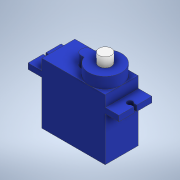
# Autodesk Inventor part: MicroServo
Saved by Autodesk Inventor 2021 (Build 250183000, 183)
## iProperties
Created: 2020-12-16
Part Number: MicroServo
Material: Generisch
Document SubType Name: Modeling
Designer: laure
Density: 1 g/cm^3
Appearance: Vorgabe
Author: laure
Autodesk Inventor part; units mm, degrees
ref_plane "YZ Plane" through (0, 0, 0) normal (1, 0, 0) x (0, 1, 0)
ref_plane "XZ Plane" through (0, 0, 0) normal (0, 1, 0) x (-1, 0, 0)
ref_plane "XY Plane" through (0, 0, 0) normal (0, 0, 1) x (1, 0, 0)
sketch "Skizze1" plane through (0, 0, 0) normal (0, 0, 1) x (1, 0, 0)
  line L0 (-11.5, 11) -> (11.5, 11)
  line L1 (11.5, 11) -> (11.5, -11)
  line L2 (11.5, -11) -> (-11.5, -11)
  line L3 (-11.5, -11) -> (-11.5, 11)
  line L4 (0, -15.4) -> (0, 15.4) projected
  line L5 (-23.1, 0) -> (23.1, 0) projected
  line L6 (-11.5, 7) -> (-16.5, 7)
  line L7 (-16.5, 7) -> (-16.5, 5)
  line L8 (-16.5, 5) -> (-11.5, 5)
  line L9 (-11.5, 5) -> (-11.5, 7)
  line L10 (11.5, 7) -> (16.5, 7)
  line L11 (16.5, 7) -> (16.5, 5)
  line L12 (16.5, 5) -> (11.5, 5)
  line L13 (11.5, 5) -> (11.5, 7)
  point P0 (0, 0)
  dimension "d0" = 23
  dimension "d1" = 22
  dimension "d2" = 16
  dimension "d3" = 2
  dimension "d4" = 5
  constraints: 24 end point, 4 parallel, 4 symmetric about line, 2 horizontal, 2 perpendicular, 1 point on line, 2 other
  measures "d0" distance between parallel lines of L1 L3
  measures "d1" distance between parallel lines of L2 L0
  measures "d2" distance between parallel lines of L8 L2
  measures "d3" distance between parallel lines of L6 L8
  measures "d4" distance between parallel lines of L7 L3
extrude "Extrusion1" add sketch "Skizze1" against normal mid plane 12 contours L0 L4 L5 L3 | L0 L1 L5 L4 | L5 L1 L2 L4 | L4 L2 L3 L5
extrude "Extrusion2" add sketch "Skizze1" along normal mid plane 12 contours L3 L8 L7 L6 | L10 L11 L12 L1
sketch "Skizze2" plane through (-11.5, 11, -6) normal (0, 1, 0) x (1, 0, 0)
  arc A0 (11.3431, -8) -> (11.3431, -4) centre (17, -6) ccw
  line L0 (0, 0) -> (23, 0) projected
  line L1 (23, 0) -> (23, -12) projected
  arc A1 (10.2601, -4) -> (10.2601, -8) centre (10.2601, -6) ccw
  line L2 (10.2601, -4) -> (11.3431, -4)
  line L3 (10.2601, -8) -> (11.3431, -8)
  point P0 (11.5, -6)
  dimension "d9" = 6
  dimension "d10" = 6
  dimension "d11" = 4
  constraints: 4 end point, 4 point on circle, 3 tangent, 2 centre point, 1 horizontal, 1 parallel
  measures "d9" distance from line of L1 A0.centre
  measures "d10" distance from line of L0 A0.centre
  measures "d11" diameter of A1
extrude "Extrusion3" add sketch "Skizze2" along normal blind 4 contours L3 A1 L2 A0
sketch "Skizze3" plane through (-16.5, 7, 6) normal (0, 1, 0) x (1, 0, 0)
  arc A0 (1.134, 5.5) -> (1.134, 6.5) centre (2, 6) ccw
  line L0 (0, 12) -> (0, 0) projected
  arc A1 (31.866, 6.5) -> (31.866, 5.5) centre (31, 6) ccw
  line L1 (33, 0) -> (33, 12) projected
  line L2 (1.134, 6.5) -> (0, 6.5)
  line L3 (1.134, 5.5) -> (0, 5.5)
  line L4 (31.866, 6.5) -> (33, 6.5)
  line L5 (33, 12) -> (33, 0) projected
  line L6 (31.866, 5.5) -> (33, 5.5)
  line L7 (-6.6, 6) -> (39.6, 6) projected
  line L8 (0, 6.5) -> (0, 5.5)
  line L9 (33, 6.5) -> (33, 5.5)
  point P0 (16.5, 6)
  dimension "d14" = 2
  dimension "d15" = 2
  dimension "d16" = 2
  dimension "d17" = 2
  dimension "d18" = 1
  constraints: 12 end point, 8 point on line, 4 point on circle, 2 centre point, 2 collinear, 2 perpendicular, 1 other
  measures "d14" diameter of A0
  measures "d15" distance from line of L0 A0.centre
  measures "d16" diameter of A1
  measures "d17" distance from line of A1.centre L1
  measures "d18" distance between parallel lines of L2 L3
extrude "Extrusion4" cut sketch "Skizze3" against normal blind 2
sketch "Skizze4" plane through (-11.5, 15, -6) normal (0, 1, 0) x (1, 0, 0)
  circle A0 centre (17, -6) radius 2.25
  line L0 (23, -6) -> (23, -12) projected
  point P0 (11.5, -6)
  dimension "d21" = 4.5
  dimension "d22" = 6
  constraints: 1 centre point
  measures "d21" diameter of A0
  measures "d22" distance from line of A0.centre L0
extrude "Extrusion5" add sketch "Skizze4" along normal blind 3.5
